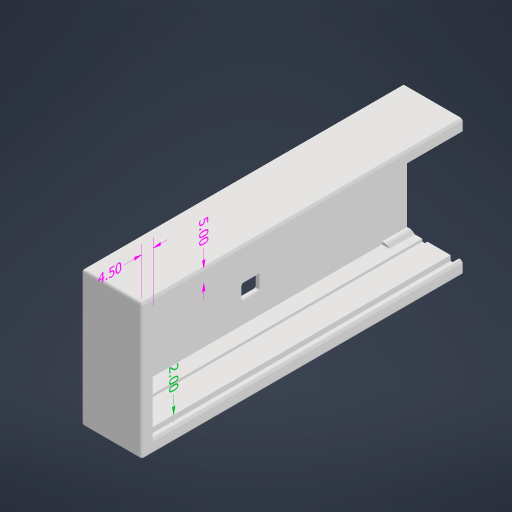
# Autodesk Inventor part: V2.0 Case
Saved by Autodesk Inventor 2023 (Build 270158000, 158)
## iProperties
Created: 2022-12-23
Part Number: V2.0 Case
Material: Generic
Document SubType Name: Modeling
Designer: User
Density: 1 g/cm^3
Appearance: Default
Author: User
Autodesk Inventor part; units mm, degrees
ref_plane "YZ Plane" through (0, 0, 0) normal (1, 0, 0) x (0, 1, 0)
ref_plane "XZ Plane" through (0, 0, 0) normal (0, 1, 0) x (-1, 0, 0)
sketch "Sketch1" plane through (0, 0, 0) normal (0, 0, 1) x (1, 0, 0)
  line L0 (0, -44.5) -> (0, 0) projected
  line L1 (0, -44.5) -> (9.25, -44.5) projected
  line L2 (9.25, 0) -> (9.25, -44.5) projected
  line L3 (0, 0) -> (9.25, 0) projected
  line L4 (-1.75, 0) -> (-1.75, -44.5) projected
  line L5 (-1.75, -44.5) -> (0, -44.5) projected
  line L6 (0, 0) -> (0, -44.5) projected
  line L7 (-1.75, 0) -> (0, 0) projected
  line L8 (-1.75, 1) -> (0, 1) projected
  line L9 (0, 0) -> (0, 1) projected
  line L10 (-1.75, 0) -> (-1.75, 1) projected
  line L11 (0, -45.5) -> (0, -44.5) projected
  line L12 (-1.75, -45.5) -> (0, -45.5) projected
  line L13 (-1.75, -45.5) -> (-1.75, -44.5) projected
  line L14 (0.15, -44.65) -> (9.4, -44.65)
  line L15 (9.4, -44.65) -> (9.4, 0.15)
  line L16 (9.4, 0.15) -> (0.15, 0.15)
  line L17 (0.15, -44.65) -> (0.15, -45.65)
  line L18 (0.15, -45.65) -> (-1.9, -45.65)
  line L19 (-1.9, -45.65) -> (-1.9, -44.65)
  line L20 (0.15, 0.15) -> (0.15, 1.15)
  line L21 (0.15, 1.15) -> (-1.9, 1.15)
  line L22 (-1.9, 1.15) -> (-1.9, 0.15)
  line L23 (-1.9, 0.15) -> (-7.9, 0.15)
  line L24 (-7.9, 0.15) -> (-7.9, -44.65)
  line L25 (-7.9, -44.65) -> (-1.9, -44.65)
  line L26 (9.4, -44.65) -> (9.4, -46.65)
  line L27 (9.4, -46.65) -> (12.725, -46.65)
  line L28 (12.725, -46.65) -> (12.725, -44.15)
  line L29 (12.725, -44.15) -> (14.225, -44.15)
  line L30 (14.225, -44.15) -> (14.225, -49.15)
  line L31 (14.225, -49.15) -> (-9.9, -49.15)
  line L32 (-9.9, -49.15) -> (-9.9, 4.65)
  line L33 (9.4, 0.15) -> (9.4, 2.15)
  line L34 (9.4, 2.15) -> (12.725, 2.15)
  line L35 (12.725, 2.15) -> (12.725, -0.35)
  line L36 (12.725, -0.35) -> (14.225, -0.35)
  line L37 (14.225, -0.35) -> (14.225, 4.65)
  line L38 (14.225, 4.65) -> (-9.9, 4.65)
  point P0 (-1.9, -45.15)
  dimension "d0" = 0.15
  dimension "d1" = 0.15
  dimension "d3" = 0.15
  dimension "d4" = 0.15
  dimension "d5" = 0.15
  dimension "d6" = 0.15
  dimension "d7" = 0.15
  dimension "d8" = 6
  dimension "d9" = 2
  dimension "d10" = 3.325
  dimension "d11" = 2.5
  dimension "d12" = 1.5
  dimension "d13" = 5
  dimension "d14" = 2
  dimension "d15" = 2.5
  dimension "d16" = 1.5
  dimension "d17" = 5
  dimension "d18" = 2
  constraints: 50 end point, 11 perpendicular, 3 collinear, 2 parallel, 2 vertical, 1 horizontal, 1 midpoint, 2 other
  measures "d0" distance between parallel lines of L1 L14
  measures "d1" distance between parallel lines of L11 L17
  measures "d3" distance between parallel lines of L9 L20
  measures "d4" distance from line of point (-1.9, -45.15) L13
  measures "d5" distance between parallel lines of L3 L16
  measures "d6" distance between parallel lines of L2 L15
  measures "d7" distance between parallel lines of L8 L21
  measures "d8" distance of L22.end L23.end
  measures "d9" distance of L14.end L26.end
  measures "d10" distance of L26.end L27.end
  measures "d11" distance of L27.end L28.end
  measures "d12" distance of L28.end L29.end
  measures "d13" distance of L29.end L30.end
  measures "d14" distance of L15.end L33.end
  measures "d15" distance of L34.end L35.end
  measures "d16" distance of L35.end L36.end
  measures "d17" distance of L36.end L37.end
  measures "d18" distance between parallel lines of L32 L24
ref_plane "Work Plane1" through (0, -44.5, -123) normal (0, 0, -1) x (0, 1, 0)
extrude "Extrusion1" add sketch "Sketch1" against normal up to surface (123 mm away) contours L14 L26 L27 L28 L29 L30 L31 L32 L38 L37 L36 L35 L34 L33 L16 L20 L21 L22 L23 L24 L25 L19 L18 L17
sketch "Sketch2" plane through (0, 0, 0) normal (0, 0, 1) x (1, 0, 0)
  line L0 (9.4, 0.15) -> (9.4, 2.15) projected
  line L1 (9.4, 2.15) -> (12.725, 2.15) projected
  line L2 (12.725, 2.15) -> (12.725, -0.35) projected
  line L3 (12.725, -0.35) -> (14.225, -0.35) projected
  line L4 (14.225, -0.35) -> (14.225, 4.65) projected
  line L5 (14.225, 4.65) -> (-9.9, 4.65) projected
  line L6 (-9.9, 4.65) -> (-9.9, -49.15) projected
  line L7 (-9.9, -49.15) -> (14.225, -49.15) projected
  line L8 (14.225, -49.15) -> (14.225, -44.15) projected
  line L9 (14.225, -44.15) -> (12.725, -44.15) projected
  line L10 (12.725, -44.15) -> (12.725, -46.65) projected
  line L11 (12.725, -46.65) -> (9.4, -46.65) projected
  line L12 (9.4, -46.65) -> (9.4, -44.65) projected
  line L13 (9.4, -44.65) -> (0.15, -44.65) projected
  line L14 (0.15, -44.65) -> (0.15, -45.65) projected
  line L15 (0.15, -45.65) -> (-1.9, -45.65) projected
  line L16 (-1.9, -45.65) -> (-1.9, -44.65) projected
  line L17 (-1.9, -44.65) -> (-7.9, -44.65) projected
  line L18 (-7.9, -44.65) -> (-7.9, 0.15) projected
  line L19 (-7.9, 0.15) -> (-1.9, 0.15) projected
  line L20 (-1.9, 0.15) -> (-1.9, 1.15) projected
  line L21 (-1.9, 1.15) -> (0.15, 1.15) projected
  line L22 (0.15, 1.15) -> (0.15, 0.15) projected
  line L23 (0.15, 0.15) -> (9.4, 0.15) projected
  line L24 (-7.9, -44.65) -> (-7.9, 0.15) projected
  line L25 (-7.9, 0.15) -> (-1.9, 0.15)
  line L26 (-1.9, 0.15) -> (-1.9, -44.65)
  line L27 (-1.9, -44.65) -> (-7.9, -44.65)
  line L28 (-7.9, -44.65) -> (-7.9, 0.15)
  line L29 (0.15, -44.65) -> (9.4, -44.65)
  line L30 (9.4, -44.65) -> (9.4, 0.15)
  line L31 (9.4, 0.15) -> (0.15, 0.15)
  line L32 (0.15, 0.15) -> (0.15, -44.65)
  line L33 (12.725, -0.35) -> (14.225, -0.35)
  line L34 (14.225, -0.35) -> (14.225, -44.15)
  line L35 (14.225, -44.15) -> (12.725, -44.15)
  line L36 (12.725, -44.15) -> (12.725, -0.35)
  point P0 (0, 0)
  constraints: 24 end point, 6 parallel, 3 horizontal, 3 perpendicular
extrude "Extrusion2" add sketch "Sketch2" along normal blind 4.5 contours L23 L22 L21 L20 L19 L18 L17 L16 L15 L14 L13 L12 L11 L10 L9 L8 L7 L6 L5 L4 L3 L2 L1 L0 | L30 L13 L32 L23 | L3 L34 L9 L36 | L26 L17 L18 L19
sketch "Sketch3" plane through (0, 0, 4.5) normal (0, 0, 1) x (1, 0, 0)
  line L0 (14.225, -49.15) -> (14.225, 4.65) projected
  line L1 (14.225, 4.65) -> (-9.9, 4.65) projected
  line L2 (-9.9, 4.65) -> (-9.9, -49.15) projected
  line L3 (-9.9, -49.15) -> (14.225, -49.15) projected
  line L4 (12.725, 2.15) -> (12.725, -46.65) projected
  line L5 (12.725, -46.65) -> (9.4, -46.65) projected
  line L6 (9.4, -46.65) -> (9.4, 2.15) projected
  line L7 (9.4, 2.15) -> (12.725, 2.15) projected
  line L8 (0.15, 1.15) -> (0.15, -45.65) projected
  line L9 (0.15, -45.65) -> (-1.9, -45.65) projected
  line L10 (-1.9, -45.65) -> (-1.9, 1.15) projected
  line L11 (-1.9, 1.15) -> (0.15, 1.15) projected
  point P0 (0, 0)
extrude "Extrusion3" add sketch "Sketch3" against normal blind 3.5 contours L8 L9 L10 L11
sketch "Sketch4" plane through (0, 0, 4.5) normal (0, 0, 1) x (1, 0, 0)
  line L0 (14.225, -49.15) -> (14.225, 4.65) projected
  line L1 (14.225, 4.65) -> (-9.9, 4.65) projected
  line L2 (-9.9, 4.65) -> (-9.9, -49.15) projected
  line L3 (-9.9, -49.15) -> (14.225, -49.15) projected
  line L4 (12.725, 2.15) -> (12.725, -46.65) projected
  line L5 (12.725, -46.65) -> (9.4, -46.65) projected
  line L6 (9.4, -46.65) -> (9.4, 2.15) projected
  line L7 (9.4, 2.15) -> (12.725, 2.15) projected
  point P0 (0, 0)
extrude "Extrusion4" add sketch "Sketch4" against normal blind 2.5 contours L4 L5 L6 L7
sketch "Sketch5" plane through (0, 0, 0) normal (0, 0, -1) x (-1, 0, 0)
  line L0 (-12.725, -0.35) -> (-14.225, -0.35) projected
  line L1 (-14.225, -44.15) -> (-14.225, -0.35) projected
  line L2 (-14.225, -44.15) -> (-12.725, -44.15) projected
  line L3 (-12.725, -0.35) -> (-12.725, -44.15) projected
  point P0 (0, 0)
extrude "Extrusion5" add sketch "Sketch5" along normal blind 0.5
sketch "Sketch6" plane through (14.225, -49.15, -123) normal (0, 0, -1) x (-1, 0, 0)
  circle A0 centre (21.325, 51) radius 1.8
  circle A1 centre (21.325, 51) radius 2.8
  line L0 (0, 53.8) -> (24.125, 53.8) projected
  line L1 (24.125, 53.8) -> (24.125, 0) projected
  circle A2 centre (21.325, 2.8) radius 1.8
  circle A3 centre (21.325, 2.8) radius 2.8
  line L2 (24.125, 0) -> (0, 0) projected
  line L3 (4.825, 51.3) -> (1.5, 51.3) projected
  line L4 (4.825, 49.3) -> (4.825, 51.3) projected
  line L5 (14.075, 49.3) -> (4.825, 49.3) projected
  line L6 (14.075, 50.3) -> (14.075, 49.3) projected
  line L7 (16.125, 50.3) -> (14.075, 50.3) projected
  line L8 (16.125, 49.3) -> (16.125, 50.3) projected
  line L9 (22.125, 49.3) -> (16.125, 49.3) projected
  line L10 (22.125, 4.5) -> (22.125, 49.3) projected
  line L11 (16.125, 4.5) -> (22.125, 4.5) projected
  line L12 (16.125, 3.5) -> (16.125, 4.5) projected
  line L13 (14.075, 3.5) -> (16.125, 3.5) projected
  line L14 (14.075, 4.5) -> (14.075, 3.5) projected
  line L15 (4.825, 4.5) -> (14.075, 4.5) projected
  line L16 (4.825, 2.5) -> (4.825, 4.5) projected
  line L17 (1.5, 2.5) -> (4.825, 2.5) projected
  line L18 (1.5, 5) -> (1.5, 2.5) projected
  line L19 (0, 5) -> (1.5, 5) projected
  line L20 (0, 0) -> (0, 5) projected
  line L21 (24.125, 0) -> (0, 0) projected
  line L22 (24.125, 53.8) -> (24.125, 0) projected
  line L23 (0, 53.8) -> (24.125, 53.8) projected
  line L24 (0, 48.8) -> (0, 53.8) projected
  line L25 (1.5, 48.8) -> (0, 48.8) projected
  line L26 (1.5, 51.3) -> (1.5, 48.8) projected
  point P0 (14.225, 49.15)
  dimension "d41" = 3.6
  dimension "d42" = 1
  dimension "d43" = 3.6
  dimension "d44" = 1
  constraints: 4 centre point, 4 tangent
  measures "d41" diameter of A0
  measures "d42" radial gap between concentric circles of A0 A1
  measures "d43" diameter of A2
  measures "d44" radial gap between concentric circles of A2 A3
extrude "Extrusion6" add sketch "Sketch6" against normal blind 10 contours A0 L9 | A0 L9 A1 L10 | L9 A0 | A0 L9 L10 A1 | L10 L11 A2 A3 | A3 L11 A2 L10 | L11 A2 | A2 L11
sketch "Sketch7" plane through (14.225, 4.65, -123) normal (0, 0, -1) x (-1, 0, 0)
  arc A0 (19.1001, -4.5) -> (22.125, -5.4833) centre (21.325, -2.8) ccw projected
  arc A1 (22.125, -48.3167) -> (19.1001, -49.3) centre (21.325, -51) ccw projected
  circle A2 centre (21.325, -2.8) radius 1.6
  circle A3 centre (21.325, -51) radius 1.6
  point P0 (14.225, -4.65)
  dimension "d47" = 3.2
  dimension "d48" = 3.2
  constraints: 2 centre point, 2 coincident
  measures "d47" diameter of A2
  measures "d48" diameter of A3
extrude "Extrusion7" cut sketch "Sketch7" against normal blind 8
chamfer "Chamfer2" distance 0.75 angle 45 3 edges at (14.225, -0.35, -61.75) (14.225, -44.15, -61.75) (14.225, -22.25, -0.5)
sketch "Sketch8" plane through (-7.9, -44.65, 0) normal (1, 0, 0) x (0, 0, -1)
  line L0 (0.5, 0.5) -> (0.5, 44.3) projected
  line L1 (123, 0.9833) -> (123, 43.8167) projected
  line L2 (124, 45.8) -> (124, 27.4772) projected
  line L3 (-2, -2) -> (-2, 46.8) projected
  line L4 (-2, 46.8) -> (-2, -2) projected
  line L5 (59.5, 12.05) -> (62.5, 12.05) construction
  line L6 (62.5, 12.05) -> (62.5, 10.55) construction
  line L7 (62.5, 10.55) -> (59.5, 10.55) construction
  line L8 (59.5, 10.55) -> (59.5, 12.05) construction
  line L9 (64.5, 14.05) -> (57.5, 14.05)
  line L10 (57.5, 14.05) -> (57.5, 8.55)
  line L11 (57.5, 8.55) -> (64.5, 8.55)
  line L12 (64.5, 8.55) -> (64.5, 14.05)
  line L13 (123, 46.8) -> (-2, 46.8) projected
  line L14 (124, 27.4772) -> (-2, 27.4772) construction
  circle A0 centre (61, 35.42) radius 2.5
  circle A1 centre (61, 41.47) radius 2.5
  point P0 (0, 44.65)
  point P1 (61, 12.05)
  point P2 (61, 27.4772)
  dimension "d61" = 3
  dimension "d62" = 1.5
  dimension "d63" = 2
  dimension "d64" = 34.75
  dimension "d65" = 5
  dimension "d66" = 5
  dimension "d67" = 6.05
  dimension "d68" = 5.33
  constraints: 18 end point, 4 parallel, 3 perpendicular, 3 vertical alignment, 2 centre point, 2 midpoint, 1 horizontal, 1 point on line, 3 other
  measures "d61" distance of L5.start L5.end
  measures "d62" distance of L7.end L5.start
  measures "d63" distance between parallel lines of L5 L9
  measures "d64" distance between parallel lines of L5 L13
  measures "d65" diameter of A0
  measures "d66" diameter of A1
  measures "d67" distance of A0.centre A1.centre
  measures "d68" distance from line of A1.centre L13
extrude "Extrusion8" cut sketch "Sketch8" against normal through all
fillet "Fillet1" radius 1 8 edges at (14.225, 4.65, -59.25) (-9.9, 4.65, -59.25) (14.225, -49.15, -59.25) (2.1625, 4.65, 4.5) (-9.9, -22.25, 4.5) (14.225, -22.25, 4.5) (2.1625, -49.15, 4.5) (-9.9, -49.15, -59.25)
fillet "Fillet2" radius 0.5 16 edges at (-7.9, -36.1, -61) (-7.9, -33.35, -64.5) (-7.9, -30.6, -61) (-7.9, -33.35, -57.5) (-9.9, -36.1, -61) (-9.9, -33.35, -64.5) (-9.9, -30.6, -61) (-9.9, -33.35, -57.5) (-8.9, -30.6, -57.5) (-8.9, -36.1, -57.5) (-8.9, -36.1, -64.5) (-8.9, -30.6, -64.5) (-7.9, -9.23, -58.5) (-9.9, -9.23, -58.5) (-9.9, -3.18, -58.5) (-7.9, -3.18, -58.5)
body "Solid1"
